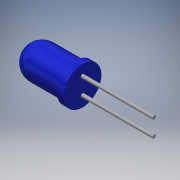
# Autodesk Inventor part: LED_5MM_BLUE_9
Saved by Autodesk Inventor 2018.3 (Build 223284000, 284)
## iProperties
Created: 2021-05-05
Part Number: LED_5MM_BLUE_9
Material: Genérico
Document SubType Name: Modeling
Designer: laguerre
Density: 8.47 g/cm^3
Appearance: Valor por defecto
Author: laguerre
Autodesk Inventor part; units mm, degrees
ref_plane "YZ Plane" through (0, 0, 0) normal (1, 0, 0) x (0, 1, 0)
ref_plane "XZ Plane" through (0, 0, 0) normal (0, 1, 0) x (-1, 0, 0)
ref_plane "XY Plane" through (0, 0, 0) normal (0, 0, 1) x (1, 0, 0)
sketch "Boceto40" plane through (0, 0, 0) normal (1, 0, 0) x (0, 1, 0)
  line L0 (0, 0) -> (0, 9.551)
  line L1 (0, 0) -> (2.9, 0)
  line L2 (2.9, 0) -> (2.9, 1)
  line L3 (2.9, 1) -> (2.5, 1)
  line L4 (2.5, 1) -> (2.5, 6.2)
  arc A0 (2.5, 6.2) -> (0, 8.7) centre (0, 6.2) ccw
  line L5 (0, 0) -> (0, 8.7)
  dimension "d373" = 5
  dimension "d374" = 5.8
  dimension "d375" = 1
  dimension "d376" = 7.7
  constraints: 12 end point, 3 perpendicular, 2 point on circle, 1 centre point, 1 collinear, 1 horizontal, 1 line through centre, 1 point on line, 1 tangent, 1 vertical
  measures "d373" diameter of L4 L0
  measures "d374" diameter of L2 L0
  measures "d375" distance of L1.end L2.end
  measures "d376" vertical distance of L2.end L5.end
revolve "Revolución14" add sketch "Boceto40" angle 360 about axis through (0, 0, 0) along (0, 0, 1)
sketch "Boceto41" plane through (0, 0, 0) normal (0, 0, -1) x (-1, 0, 0)
  circle A0 centre (0, 1.27) radius 0.27
  circle A1 centre (0, -1.27) radius 0.27
  point P0 (0, 0)
  dimension "d378" = 2.54
  dimension "d379" = 1.27
  dimension "d380" = 0.54
  constraints: 2 centre point, 2 vertical alignment, 1 equal radius
  measures "d378" distance of A0.centre A1.centre
  measures "d379" distance of point (0, 0) A0.centre
  measures "d380" diameter of A1
extrude "Extrusión13" add sketch "Boceto41" along normal blind 11
